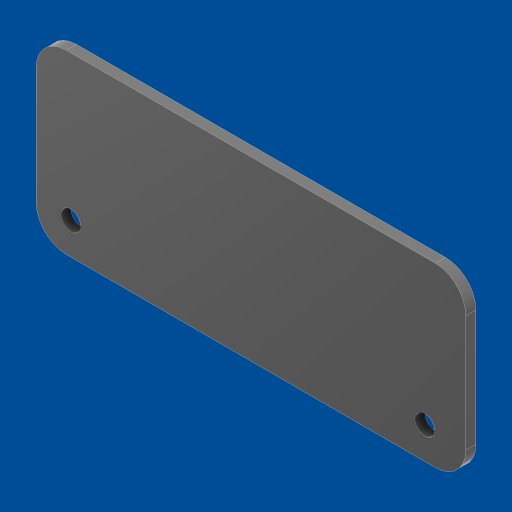
# Autodesk Inventor part: CASE_1
Saved by Autodesk Inventor 2023.2 (Build 272271000, 271)
## iProperties
Created: 2023-06-14
Part Number: CASE_1
Material: Generic
Document SubType Name: Modeling
Designer: samdi
Density: 1 g/cm^3
Appearance: Smooth - Black
Author: samdi
Autodesk Inventor part; units mm, degrees
ref_plane "YZ Plane" through (0, 0, 0) normal (1, 0, 0) x (0, 1, 0)
ref_plane "XZ Plane" through (0, 0, 0) normal (0, 1, 0) x (-1, 0, 0)
ref_plane "XY Plane" through (0, 0, 0) normal (0, 0, 1) x (1, 0, 0)
sketch "Sketch1" plane through (0, 0, 0) normal (0, 0, 1) x (1, 0, 0)
  line L0 (-35.8578, -17.234) -> (37.1422, -17.234)
  arc A0 (37.1422, -17.234) -> (43.1422, -11.234) centre (37.1422, -11.234) ccw
  line L1 (43.1422, -11.234) -> (43.1422, 11.766)
  arc A1 (43.1422, 11.766) -> (37.1422, 17.766) centre (37.1422, 11.766) ccw
  line L2 (37.1422, 17.766) -> (-35.8578, 17.766)
  arc A2 (-35.8578, 17.766) -> (-41.8578, 11.766) centre (-35.8578, 11.766) ccw
  line L3 (-41.8578, 11.766) -> (-41.8578, -11.234)
  arc A3 (-41.8578, -11.234) -> (-35.8578, -17.234) centre (-35.8578, -11.234) ccw
  arc A4 (41.1422, 12.766) -> (38.1422, 15.766) centre (38.1422, 12.766) ccw
  line L4 (41.1422, 12.766) -> (41.1422, -12.234)
  arc A5 (38.1422, -15.234) -> (41.1422, -12.234) centre (38.1422, -12.234) ccw
  line L5 (38.1422, -15.234) -> (-36.8578, -15.234)
  arc A6 (-39.8578, -12.234) -> (-36.8578, -15.234) centre (-36.8578, -12.234) ccw
  line L6 (-39.8578, -12.234) -> (-39.8578, 12.766)
  arc A7 (-36.8578, 15.766) -> (-39.8578, 12.766) centre (-36.8578, 12.766) ccw
  line L7 (-36.8578, 15.766) -> (38.1422, 15.766)
  point P0 (0, 0)
  point P1 (0.6422, 0.266)
  constraints: 16 end point, 16 point on circle, 8 centre point
extrude "Extrusion1" add sketch "Sketch1" along normal blind 2 contours A3 L3 A2 L2 A1 L1 A0 L0 | L4 A5 L5 A6 L6 A7 L7 A4
sketch "Sketch2" plane through (0, 0, 2) normal (0, 0, 1) x (1, 0, 0)
  line L0 (0, 0) -> (-35, 0)
  line L1 (-35, 0) -> (-35, -11)
  line L2 (-35, -11) -> (35, -11)
  line L3 (-35, -9) -> (-35, -9)
  line L4 (-33, -11) -> (-33, -11)
  line L5 (-35, -13) -> (-35, -13)
  line L6 (-37, -11) -> (-37, -11)
  line L7 (-37, -9) -> (-33, -13) construction
  line L8 (-33, -9) -> (-37, -13) construction
  line L9 (35, -9) -> (35, -9)
  line L10 (37, -11) -> (37, -11)
  line L11 (35, -13) -> (35, -13)
  line L12 (33, -11) -> (33, -11)
  line L13 (33, -9) -> (37, -13) construction
  line L14 (37, -9) -> (33, -13) construction
  arc A0 (35, -9) -> (33, -11) centre (35, -11) ccw
  arc A1 (37, -11) -> (35, -9) centre (35, -11) ccw
  arc A2 (33, -11) -> (35, -13) centre (35, -11) ccw
  arc A3 (35, -13) -> (37, -11) centre (35, -11) ccw
  arc A4 (-33, -11) -> (-35, -9) centre (-35, -11) ccw
  arc A5 (-35, -13) -> (-33, -11) centre (-35, -11) ccw
  arc A6 (-37, -11) -> (-35, -13) centre (-35, -11) ccw
  arc A7 (-35, -9) -> (-37, -11) centre (-35, -11) ccw
  dimension "d2" = 35
  dimension "d3" = 11
  dimension "d4" = 70
  dimension "d5" = 4
  dimension "d6" = 4
  dimension "d7" = 4
  dimension "d8" = 4
  dimension "d9" = 2
  constraints: 30 end point, 16 point on circle, 16 point on line, 16 tangent, 8 centre point, 7 equal radius, 4 midpoint, 4 parallel, 4 perpendicular, 3 horizontal
  measures "d2" distance of L0.start L0.end
  measures "d3" distance of L0.end L1.end
  measures "d4" distance of L1.end L2.end
  measures "d5" distance of L7.end L8.end
  measures "d6" distance of L8.start L7.end
  measures "d7" distance of L13.end L14.end
  measures "d8" distance of L14.start L13.end
  measures "d9" radius of A0
extrude "Extrusion2" cut sketch "Sketch2" against normal blind 2
body "Solid1"
